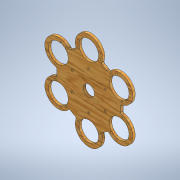
# Autodesk Inventor part: AmmoHolder
Saved by Autodesk Inventor 2020.2 (Build 242310000, 310)
## iProperties
Created: 2019-11-06
Part Number: AmmoHolder
Material: Plywood, Finish
Document SubType Name: Modeling
Designer: Paul Lefeuvre
Density: 0.552 g/cm^3
Appearance: Plywood - New
Mass: 279.601 g
Surface Area: 1409.01 cm^2
Volume: 506.524 cm^3
Author: Paul Lefeuvre
Autodesk Inventor part; units mm, degrees
ref_plane "YZ Plane" through (0, 0, 0) normal (1, 0, 0) x (0, 1, 0)
ref_plane "XZ Plane" through (0, 0, 0) normal (0, 1, 0) x (-1, 0, 0)
ref_plane "XY Plane" through (0, 0, 0) normal (0, 0, 1) x (1, 0, 0)
sketch "Sketch3" plane through (0, 0, 0) normal (0, 0, 1) x (1, 0, 0)
  circle A0 centre (0, 0) radius 175 construction
  circle A1 centre (0, 136.9) radius 37.5 construction
  circle A2 centre (0, 136.9) radius 38.1
  line L0 (0, 0) -> (0, 212.7207) construction
  arc A3 (50.163, 119.485) -> (-50.163, 119.485) centre (0, 136.9) ccw
  arc A4 (-52.7754, 113.3126) -> (-50.163, 119.485) centre (-54.8865, 117.8451) ccw
  arc A5 (50.163, 119.485) -> (52.7754, 113.3126) centre (54.8865, 117.8451) ccw
  circle A6 centre (0, 0) radius 12.5
  circle A7 centre (0, 0) radius 21 construction
  circle A8 centre (-118.5589, 68.45) radius 38.1
  arc A9 (-78.3955, 103.1849) -> (-128.5585, 16.3001) centre (-118.5589, 68.45) ccw
  arc A10 (-124.5193, 10.9515) -> (-128.5585, 16.3001) centre (-129.5001, 11.3895) ccw
  arc A11 (-78.3955, 103.1849) -> (-71.7439, 102.3612) centre (-74.6137, 106.4556) ccw
  circle A12 centre (-118.5589, -68.45) radius 38.1
  arc A13 (-128.5585, -16.3001) -> (-78.3955, -103.1849) centre (-118.5589, -68.45) ccw
  arc A14 (-71.7439, -102.3612) -> (-78.3955, -103.1849) centre (-74.6137, -106.4556) ccw
  arc A15 (-128.5585, -16.3001) -> (-124.5193, -10.9515) centre (-129.5001, -11.3895) ccw
  circle A16 centre (0, -136.9) radius 38.1
  arc A17 (-50.163, -119.485) -> (50.163, -119.485) centre (0, -136.9) ccw
  arc A18 (52.7754, -113.3126) -> (50.163, -119.485) centre (54.8865, -117.8451) ccw
  arc A19 (-50.163, -119.485) -> (-52.7754, -113.3126) centre (-54.8865, -117.8451) ccw
  circle A20 centre (118.5589, -68.45) radius 38.1
  arc A21 (78.3955, -103.1849) -> (128.5585, -16.3001) centre (118.5589, -68.45) ccw
  arc A22 (124.5193, -10.9515) -> (128.5585, -16.3001) centre (129.5001, -11.3895) ccw
  arc A23 (78.3955, -103.1849) -> (71.7439, -102.3612) centre (74.6137, -106.4556) ccw
  circle A24 centre (118.5589, 68.45) radius 38.1
  arc A25 (128.5585, 16.3001) -> (78.3955, 103.1849) centre (118.5589, 68.45) ccw
  arc A26 (71.7439, 102.3612) -> (78.3955, 103.1849) centre (74.6137, 106.4556) ccw
  arc A27 (128.5585, 16.3001) -> (124.5193, 10.9515) centre (129.5001, 11.3895) ccw
  arc A28 (-52.7754, 113.3126) -> (-71.7439, 102.3612) centre (0, 0) ccw
  arc A29 (71.7439, 102.3612) -> (52.7754, 113.3126) centre (0, 0) ccw
  arc A30 (124.5193, -10.9515) -> (124.5193, 10.9515) centre (0, 0) ccw
  arc A31 (52.7754, -113.3126) -> (71.7439, -102.3612) centre (0, 0) ccw
  arc A32 (-71.7439, -102.3612) -> (-52.7754, -113.3126) centre (0, 0) ccw
  arc A33 (-124.5193, 10.9515) -> (-124.5193, -10.9515) centre (0, 0) ccw
  circle A34 centre (0, 0) radius 74.4
  circle A35 centre (0, 74.4) radius 3.9
  circle A36 centre (0, 0) radius 74.4
  circle A37 centre (-64.4323, 37.2) radius 3.9
  circle A38 centre (0, 0) radius 74.4
  circle A39 centre (-64.4323, -37.2) radius 3.9
  circle A40 centre (0, 0) radius 74.4
  circle A41 centre (0, -74.4) radius 3.9
  circle A42 centre (0, 0) radius 74.4
  circle A43 centre (64.4323, -37.2) radius 3.9
  circle A44 centre (0, 0) radius 74.4
  circle A45 centre (64.4323, 37.2) radius 3.9
  circle A46 centre (0, 0) radius 21.6
  circle A47 centre (41.5415, 124.9) radius 3.3
  line L1 (0, 136.9) -> (41.5415, 124.9) construction
  circle A48 centre (41.5415, 148.9) radius 3.3
  line L2 (0, 136.9) -> (41.5415, 148.9) construction
  line L3 (41.5415, 124.9) -> (41.5415, 148.9) construction
  circle A49 centre (-41.5415, 124.9) radius 3.3
  circle A50 centre (-41.5415, 148.9) radius 3.3
  circle A51 centre (-149.7219, 38.474) radius 3.3
  circle A52 centre (-128.9373, 26.474) radius 3.3
  circle A53 centre (-108.1804, 110.426) radius 3.3
  circle A54 centre (-87.3958, 98.426) radius 3.3
  circle A55 centre (-108.1804, -110.426) radius 3.3
  circle A56 centre (-87.3958, -98.426) radius 3.3
  circle A57 centre (-149.7219, -38.474) radius 3.3
  circle A58 centre (-128.9373, -26.474) radius 3.3
  circle A59 centre (41.5415, -148.9) radius 3.3
  circle A60 centre (41.5415, -124.9) radius 3.3
  circle A61 centre (-41.5415, -148.9) radius 3.3
  circle A62 centre (-41.5415, -124.9) radius 3.3
  circle A63 centre (149.7219, -38.474) radius 3.3
  circle A64 centre (128.9373, -26.474) radius 3.3
  circle A65 centre (108.1804, -110.426) radius 3.3
  circle A66 centre (87.3958, -98.426) radius 3.3
  circle A67 centre (108.1804, 110.426) radius 3.3
  circle A68 centre (87.3958, 98.426) radius 3.3
  circle A69 centre (149.7219, 38.474) radius 3.3
  circle A70 centre (128.9373, 26.474) radius 3.3
  point P0 (-34.2525, 120.2155)
  point P1 (34.2525, 120.2155)
  point P2 (-121.2359, 30.4442)
  point P3 (-86.9834, 89.7713)
  point P4 (-86.9834, -89.7713)
  point P5 (-121.2359, -30.4442)
  point P6 (34.2525, -120.2155)
  point P7 (-34.2525, -120.2155)
  point P8 (121.2359, -30.4442)
  point P9 (86.9834, -89.7713)
  point P10 (86.9834, 89.7713)
  point P11 (121.2359, 30.4442)
  dimension "d14" = 148.8
  dimension "d0" = 350
  dimension "d1" = 75
  dimension "d2" = 0.6
  dimension "d4" = 15
  dimension "d5" = 5
  dimension "d7" = 25
  dimension "d8" = 42
  dimension "d11" = 360
  dimension "d15" = 7.8
  dimension "d18" = 360
  dimension "d22" = 0.6
  dimension "d23" = 125
  dimension "d24" = 6.6
  dimension "d26" = 43.24
  dimension "d27" = 6.6
  dimension "d28" = 43.24
  dimension "d29" = 24
  dimension "d32" = 360
  constraints: 65 centre point, 60 point on circle, 8 end point, 5 coincident, 3 tangent, 2 point on line, 2 symmetric about line, 2 vertical, 2 vertical alignment, 1 equal radius, 171 other
  measures "d0" diameter of A0
  measures "d1" diameter of A1
  measures "d2" radial gap between concentric circles of A1 A2
  measures "d4" radial gap between concentric circles of A2 A3
  measures "d5" radius of A4
  measures "d7" diameter of A6
  measures "d8" diameter of A7
  measures "d15" diameter of A35
  measures "d22" radial gap between concentric circles of A7 A46
  measures "d23" radius of A29
  measures "d24" diameter of A47
  measures "d26" distance of L1.start L1.end
  measures "d27" diameter of A48
  measures "d28" distance of L1.start L2.end
  measures "d29" distance of L1.end L2.end
extrude "Extrusion1" add sketch "Sketch3" along normal blind 9 contours A5 A29 A26 A25 A27 A30 A22 A21 A23 A31 A18 A17 A19 A32 A14 A13 A15 A33 A10 A9 A11 A28 A4 A3 | A34 A43 A41 A39 A37 A35 A45
body "Solid1"
